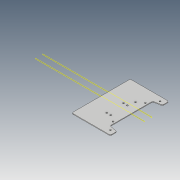
# Autodesk Inventor part: testPlate
Saved by Autodesk Inventor 2018 (Build 220112000, 112)
## iProperties
Created: 2020-01-17
Part Number: testPlate
Material: Generic
Document SubType Name: Modeling
Designer: anirudh.bali
Density: 1 g/cm^3
Appearance: Default
Author: anirudh.bali
Autodesk Inventor part; units mm, degrees
ref_plane "YZ Plane" through (0, 0, 0) normal (1, 0, 0) x (0, 1, 0)
ref_plane "XZ Plane" through (0, 0, 0) normal (0, 1, 0) x (-1, 0, 0)
ref_plane "XY Plane" through (0, 0, 0) normal (0, 0, 1) x (1, 0, 0)
sketch "Sketch1" plane through (0, 0, 0) normal (0, 1, 0) x (-1, 0, 0)
  line L0 (10.16, 0) -> (218.44, 0)
  line L1 (218.44, -165.1) -> (10.16, -165.1)
  circle A0 centre (218.44, -25.4) radius 1.75
  circle A1 centre (218.44, -82.55) radius 1.75
  circle A2 centre (218.44, -139.7) radius 1.75
  circle A3 centre (10.16, -25.4) radius 1.75
  circle A4 centre (10.16, -82.55) radius 1.75
  circle A5 centre (10.16, -139.7) radius 1.75
  line L2 (218.44, 0) -> (228.6, 0)
  line L3 (228.6, 0) -> (228.6, -165.1)
  line L4 (228.6, -165.1) -> (218.44, -165.1)
  line L5 (10.16, 0) -> (0, 0)
  line L6 (0, 0) -> (0, -165.1)
  line L7 (0, -165.1) -> (10.16, -165.1)
  dimension "d18" = 3.5
  dimension "d19" = 3.5
  dimension "d20" = 3.5
  dimension "d21" = 3.5
  dimension "d22" = 3.5
  dimension "d23" = 3.5
  dimension "d24" = 10.16
  constraints: 16 end point, 6 centre point, 3 horizontal, 2 collinear, 2 perpendicular, 1 parallel, 1 point on line
  measures "d18" diameter of A0
  measures "d19" diameter of A1
  measures "d20" diameter of A2
  measures "d21" diameter of A3
  measures "d22" diameter of A4
  measures "d23" diameter of A5
  measures "d24" distance of L0.end L2.end
extrude "Extrusion2" add sketch "Sketch1" along normal blind 1.5875
fillet "Fillet2" radius 3.175 4 edges at (0, 0.7937, 0) (0, 0.7937, -165.1) (-228.6, 0.7937, -165.1) (-228.6, 0.7937, 0)
sketch "Sketch2" plane through (0, 1.5875, 0) normal (0, 1, 0) x (1, 0, 0)
  line L0 (0, 161.925) -> (0, 3.175) projected
  line L1 (-228.6, 0) -> (0, 0)
  line L2 (0, 0) -> (0, 15.24)
  line L3 (0, 15.24) -> (-228.6, 15.24)
  line L4 (-228.6, 15.24) -> (-228.6, 0)
  line L5 (-228.6, 165.1) -> (0, 165.1)
  line L6 (0, 165.1) -> (0, 149.86)
  line L7 (0, 149.86) -> (-228.6, 149.86)
  line L8 (-228.6, 149.86) -> (-228.6, 165.1)
  dimension "d28" = 15.24
  dimension "d30" = 15.24
  constraints: 16 end point, 4 parallel, 2 horizontal, 2 perpendicular, 2 point on line
  measures "d28" distance of L2.end L1.end
  measures "d30" distance of L5.end L6.end
extrude "Extrusion3" cut sketch "Sketch2" against normal blind 1.5875
fillet "Fillet3" radius 3.175 4 edges at (-228.6, 0.7937, -15.24) (0, 0.7937, -15.24) (0, 0.7937, -149.86) (-228.6, 0.7937, -149.86)
sketch "Sketch3" plane through (0, 1.5875, 0) normal (0, 1, 0) x (1, 0, 0)
  line L0 (-19.05, 82.55) -> (-19.05, 131.6)
  line L1 (-19.05, 131.6) -> (0, 135.41)
  line L2 (-19.05, 82.55) -> (-19.05, 33.5)
  line L3 (-19.05, 33.5) -> (0, 29.69)
  line L4 (0, 135.41) -> (0, 29.69)
  point P0 (0, 0)
  constraints: 10 end point
extrude "Extrusion5" cut sketch "Sketch3" against normal blind 25.4
fillet "Fillet4" radius 3.175 4 edges at (0, 0.7937, -29.69) (-19.05, 0.7937, -33.5) (0, 0.7937, -135.41) (-19.05, 0.7937, -131.6)
ref_plane "Work Plane4" through (-3.175, 1.5875, -99.3521) normal (0, 0, -1) x (-1, 0, 0)
ref_plane "Work Plane1" through (-3.175, 1.5875, -82.55) normal (0, 0, -1) x (-1, 0, 0)
sketch "Sketch4" plane through (0, 1.5875, 0) normal (0, 1, 0) x (1, 0, 0)
  line L0 (-19.05, 36.1029) -> (-19.05, 128.9971) projected
  circle A0 centre (-24.05, 45.3771) radius 1.75
  circle A1 centre (-24.05, 119.7229) radius 1.75
  point P0 (0, 0)
  dimension "d50" = 3.5
  dimension "d51" = 3.5
  constraints: 2 centre point
  measures "d50" diameter of A0
  measures "d51" diameter of A1
extrude "Extrusion6" cut sketch "Sketch4" against normal blind 25.4
sketch "Sketch5" plane through (0, 1.5875, 0) normal (0, 1, 0) x (1, 0, 0)
  line L0 (-3.175, 15.24) -> (-225.425, 15.24) projected
  circle A0 centre (-39.7764, 94.0054) radius 1.75
  circle A1 centre (-48.6664, 94.0054) radius 1.75
  circle A2 centre (-48.6664, 55.626) radius 1.75
  circle A3 centre (-39.7764, 55.626) radius 1.75
  point P0 (0, 0)
  dimension "d62" = 3.5
  dimension "d63" = 3.5
  dimension "d67" = 3.5
  dimension "d68" = 3.5
  constraints: 4 centre point
  measures "d62" diameter of A0
  measures "d63" diameter of A1
  measures "d67" diameter of A2
  measures "d68" diameter of A3
extrude "Extrusion7" cut sketch "Sketch5" against normal blind 25.4
sketch "Sketch6" plane through (0, 1.5875, 0) normal (0, 1, 0) x (1, 0, 0)
  line L0 (-19.05, 36.1029) -> (-19.05, 128.9971) projected
  circle A0 centre (-36.83, 109.8042) radius 1.75
  point P0 (0, 0)
  dimension "d71" = 3.5
  constraints: 1 centre point
  measures "d71" diameter of A0
extrude "Extrusion8" cut sketch "Sketch6" against normal blind 25.4
sketch "Sketch7" plane through (0, 1.5875, 0) normal (0, 1, 0) x (1, 0, 0)
  line L0 (0, 27.0871) -> (0, 18.415) projected
  line L1 (-88.9, 3.8743) -> (-239.1075, 3.8743)
  line L2 (-239.1075, 3.8743) -> (-239.1075, 171.038)
  line L3 (-239.1075, 171.038) -> (-88.9, 171.038)
  line L4 (-88.9, 3.8743) -> (-88.9, 171.038)
  point P0 (0, 0)
  constraints: 8 end point, 1 horizontal, 1 parallel, 1 perpendicular
extrude "Extrusion9" cut sketch "Sketch7" against normal blind 25.4
fillet "Fillet6" radius 3.175 2 edges at (-88.9, 0.7937, -15.24) (-88.9, 0.7937, -149.86)
body "Solid2"
